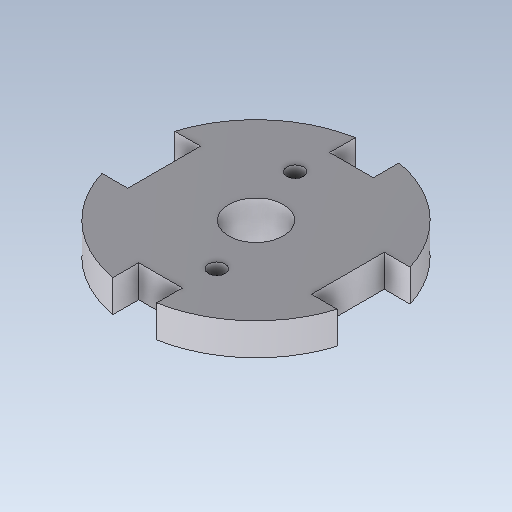
# Autodesk Inventor part: 555_Cap
Saved by Autodesk Inventor 2021 (Build 250183000, 183)
## iProperties
Created: 2021-08-07
Part Number: 555_Cap
Material: 鉄、鋳鉄
Document SubType Name: Modeling
Designer: Hagihara Yuya
Density: 7.15 g/cm^3
Appearance: 鋼
Author: Hagihara Yuya
Autodesk Inventor part; units mm, degrees
ref_plane "YZ Plane" through (0, 0, 0) normal (1, 0, 0) x (0, 1, 0)
ref_plane "XZ Plane" through (0, 0, 0) normal (0, 1, 0) x (-1, 0, 0)
ref_plane "XY Plane" through (0, 0, 0) normal (0, 0, 1) x (1, 0, 0)
sketch "スケッチ1" plane through (0, 0, 0) normal (0, 0, 1) x (1, 0, 0)
  circle A0 centre (0, 0) radius 16.9
  line L0 (-3, 13.1) -> (3, 13.1)
  line L1 (3, 13.1) -> (3, 16.9)
  line L2 (3, 16.9) -> (-3, 16.9)
  line L3 (-3, 16.9) -> (-3, 13.1)
  line L4 (-12.6, 5) -> (-16.9, 5)
  line L5 (-16.9, 5) -> (-16.9, -5)
  line L6 (-16.9, -5) -> (-12.6, -5)
  line L7 (-12.6, -5) -> (-12.6, 5)
  line L8 (16.9, 0) -> (-16.9, 0) construction
  line L9 (0, 16.9) -> (0, -16.9) construction
  line L10 (-3, -13.1) -> (3, -13.1)
  line L11 (3, -13.1) -> (3, -16.9)
  line L12 (3, -16.9) -> (-3, -16.9)
  line L13 (-3, -16.9) -> (-3, -13.1)
  line L14 (12.6, 5) -> (16.9, 5)
  line L15 (16.9, 5) -> (16.9, -5)
  line L16 (16.9, -5) -> (12.6, -5)
  line L17 (12.6, -5) -> (12.6, 5)
  point P0 (-12.6, 0)
  point P1 (0, 13.1)
  point P2 (-3, 16.6316)
  point P3 (-16.1434, 5)
  point P4 (-16.1434, -5)
  point P5 (-3, -16.6316)
  point P6 (3, -16.6316)
  point P7 (16.1434, -5)
  point P8 (16.1434, 5)
  point P9 (3, 16.6316)
  dimension "d0" = 33.8
  dimension "d1" = 6
  dimension "d2" = 10
  dimension "d3" = 3.8
  dimension "d4" = 4.3
  constraints: 36 end point, 8 symmetric about line, 4 midpoint, 4 parallel, 3 horizontal, 2 perpendicular, 2 point on circle, 2 tangent, 1 centre point, 1 coincident, 1 horizontal alignment, 1 vertical, 1 vertical alignment
  measures "d0" diameter of A0
  measures "d1" distance of L0.start L0.end
  measures "d2" distance of L6.end L4.start
  measures "d3" distance of L2.end L0.start
  measures "d4" distance of L5.end L6.end
extrude "押し出し1" add sketch "スケッチ1" along normal blind 4.4 contours L14 L17 L16 A0 L11 L10 L13 L6 L7 L4 L3 L0 L1
sketch "スケッチ2" plane through (0, 0, 0) normal (0, 0, -1) x (-1, 0, 0)
  circle A0 centre (0, 0) radius 15
  line L0 (12.8814, 7.6856) -> (10.9, 5.7042)
  line L1 (10.9, 5.7042) -> (10.9, -5.7042)
  line L2 (10.9, -5.7042) -> (12.8814, -7.6856)
  line L3 (12.6, 5) -> (12.6, -5) projected
  line L4 (15, 0) -> (-15, 0) construction
  line L5 (-6.0361, 13.7319) -> (-3.7042, 11.4)
  line L6 (-3.7042, 11.4) -> (3.7042, 11.4)
  line L7 (3.7042, 11.4) -> (6.0361, 13.7319)
  line L8 (0, 15) -> (0, -15) construction
  line L9 (-3, 13.1) -> (3, 13.1) projected
  line L10 (-12.8814, 7.6856) -> (-10.9, 5.7042)
  line L11 (-10.9, 5.7042) -> (-10.9, -5.7042)
  line L12 (-10.9, -5.7042) -> (-12.8814, -7.6856)
  line L13 (-6.0361, -13.7319) -> (-3.7042, -11.4)
  line L14 (-3.7042, -11.4) -> (3.7042, -11.4)
  line L15 (3.7042, -11.4) -> (6.0361, -13.7319)
  point P0 (-12.8814, 7.6856)
  point P1 (-12.8814, -7.6856)
  point P2 (-6.0361, -13.7319)
  point P3 (6.0361, -13.7319)
  dimension "d7" = 30
  dimension "d8" = 1.7
  dimension "d9" = 135
  dimension "d10" = 1.7
  dimension "d11" = 1.7
  dimension "d12" = 1.7
  dimension "d13" = 135
  constraints: 28 end point, 8 symmetric about line, 2 coincident, 2 horizontal, 2 midpoint, 2 vertical, 12 other
  measures "d8" distance between parallel lines of L3 L1
  measures "d9" angle of L1 L2
  measures "d10" distance from line of L3.end L2
  measures "d11" distance between parallel lines of L9 L6
  measures "d12" distance from line of L9.end L7
  measures "d13" angle of L6 L7
extrude "押し出し2" add sketch "スケッチ2" along normal blind 1.1 contours L0 L1 L2 A0 L15 L14 L13 L12 L11 L10 L5 L6 L7
sketch "スケッチ3" plane through (0, 0, -1.1) normal (0, 0, -1) x (-1, 0, 0)
  circle A0 centre (0, 0) radius 5.1
  dimension "d16" = 10.2
  constraints: 1 centre point, 1 coincident
  measures "d16" diameter of A0
extrude "押し出し3" add sketch "スケッチ3" along normal blind 3
sketch "スケッチ4" plane through (0, 0, -4.1) normal (0, 0, -1) x (-1, 0, 0)
  point P0 (0, 0)
  point P1 (0, 0)
  constraints: 1 coincident
hole "穴1" at (0, 0, -4.1) direction (0, 0, 1) diameter 7.5 end through all
fillet "フィレット1" radius 1.1 16 edges at (-11.8907, 6.6949, -1.1) (-9.9301, 11.2424, -1.1) (-4.8701, 12.566, -1.1) (0, 11.4, -1.1) (4.8701, 12.566, -1.1) (9.9301, 11.2424, -1.1) (11.8907, 6.6949, -1.1) (10.9, 0, -1.1) (11.8907, -6.6949, -1.1) (9.9301, -11.2424, -1.1) (4.8701, -12.566, -1.1) (0, -11.4, -1.1) (-4.8701, -12.566, -1.1) (-9.9301, -11.2424, -1.1) (-11.8907, -6.6949, -1.1) (-10.9, 0, -1.1)
chamfer "面取り1" distance 1.5 angle 10 1 edges at (5.1, 0, -4.1) measured on face at (-5.0835, -0.4104, -3.1)
sketch "スケッチ5" plane through (0, 0, -1.1) normal (0, 0, -1) x (-1, 0, 0)
  line L0 (-3.0782, -8.4572) -> (3.0782, 8.4572)
  line L1 (0, -23.2842) -> (0, 23.2842) projected
  point P0 (0, 0)
  point P1 (0, 0)
  dimension "d30" = 18
  dimension "d31" = 20
  constraints: 2 end point, 1 coincident, 1 midpoint
  measures "d30" distance of L0.start L0.end
  measures "d31" angle of L1 L0
hole "穴2" at (-3.0782, 8.4572, -1.1) at (3.0782, -8.4572, -1.1) direction (0, 0, 1) diameter 2.3 end through all
fillet "フィレット2" radius 0.5 2 edges at (3.0782, -9.6072, -1.1) (-3.0782, 7.3072, -1.1)
